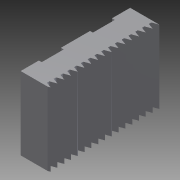
# Autodesk Inventor part: rack2
Saved by Autodesk Inventor 2011 (Build 150239000, 239)
## iProperties
Created: 2011-11-27
Part Number: rack2
Document SubType Name: Modeling
Designer: Tom
Density: 1 g/cm^3
Author: Tom
Autodesk Inventor part; units mm, degrees
ref_plane "YZ Plane" through (0, 0, 0) normal (1, 0, 0) x (0, 1, 0)
ref_plane "XZ Plane" through (0, 0, 0) normal (0, 1, 0) x (-1, 0, 0)
ref_plane "XY Plane" through (0, 0, 0) normal (0, 0, 1) x (1, 0, 0)
sketch "Sketch1" plane through (0, 0, 0) normal (0, 0, 1) x (1, 0, 0)
  line L0 (-0.515, 0.509) -> (-4.515, 0.509)
  line L1 (-4.515, -14.491) -> (-0.515, -14.491)
  line L2 (-0.515, -14.491) -> (-0.515, 0.509)
  line L3 (-4.515, -1.991) -> (-4.126, -1.991)
  line L4 (-4.126, -1.991) -> (-4.126, -4.981)
  line L5 (-4.126, -4.981) -> (-4.515, -4.981)
  line L6 (-4.515, -4.981) -> (-4.515, -1.991)
  line L7 (-4.515, -8.981) -> (-4.126, -8.981)
  line L8 (-4.126, -8.981) -> (-4.126, -11.991)
  line L9 (-4.126, -11.991) -> (-4.515, -11.991)
  line L10 (-4.515, -11.991) -> (-4.515, -8.981)
  line L11 (-4.515, 0.509) -> (-4.515, -1.991)
  line L12 (-4.515, -4.981) -> (-4.515, -14.491)
  point P0 (0, 0)
  dimension "d0" = 4
  dimension "d1" = 15
  dimension "d2" = 0.389
  dimension "d3" = 2.99
  dimension "d4" = 4
  dimension "d5" = 2.5
  dimension "d6" = 3.01
  constraints: 26 end point, 8 parallel, 4 perpendicular, 3 horizontal, 1 point on line
  measures "d0" distance of L1.start L1.end
  measures "d1" distance of L1.end L0.start
  measures "d2" distance of L3.start L3.end
  measures "d3" distance of L3.end L4.end
  measures "d4" distance between parallel lines of L7 L5
  measures "d5" distance between parallel lines of L3 L0
  measures "d6" distance of L7.end L8.end
extrude "Extrusion1" add sketch "Sketch1" along normal blind 10 contours L2 L1 L12 L9 L8 L7 L5 L4 L3 L11 L0
sketch "Sketch6" plane through (0, 0, 10) normal (0, 0, 1) x (1, 0, 0)
  line L0 (-0.515, 0.509) -> (-0.515, -14.491) projected
  line L1 (-0.515, -0.4166) -> (-1.3203, -0.1235)
  line L2 (-1.3203, -0.1235) -> (-1.3203, 0.0462)
  line L3 (-1.3203, 0.2159) -> (-0.515, 0.509)
  line L4 (-1.3203, 0.2159) -> (-1.3203, 0.0462)
  line L5 (-0.515, 0.509) -> (-0.515, -0.4166)
  line L6 (-0.412, -0.4191) -> (-1.6665, -0.4191) construction
  line L7 (-1.3203, -1.0542) -> (-0.515, -1.3473)
  line L8 (-0.515, -1.3473) -> (-0.515, -0.4216)
  line L9 (-1.3203, -1.0542) -> (-1.3203, -0.8845)
  line L10 (-1.3203, -0.7148) -> (-1.3203, -0.8845)
  line L11 (-0.515, -0.4216) -> (-1.3203, -0.7148)
  line L12 (-0.1629, -1.3498) -> (-1.5742, -1.3498) construction
  line L13 (-1.3203, -2.9154) -> (-0.515, -3.2085)
  line L14 (-0.515, -3.2085) -> (-0.515, -2.2829)
  line L15 (-1.3203, -2.9154) -> (-1.3203, -2.7457)
  line L16 (-1.3203, -2.576) -> (-1.3203, -2.7457)
  line L17 (-0.515, -2.2829) -> (-1.3203, -2.576)
  line L18 (-1.3203, -1.6454) -> (-0.515, -1.3523)
  line L19 (-0.515, -1.3523) -> (-0.515, -2.2779)
  line L20 (-1.3203, -1.6454) -> (-1.3203, -1.8151)
  line L21 (-1.3203, -1.9848) -> (-1.3203, -1.8151)
  line L22 (-0.515, -2.2779) -> (-1.3203, -1.9848)
  line L23 (-0.071, -3.211) -> (-1.4404, -3.211) construction
  line L24 (-1.3203, -6.6379) -> (-0.515, -6.9311)
  line L25 (-0.515, -6.9311) -> (-0.515, -6.0054)
  line L26 (-1.3203, -6.6379) -> (-1.3203, -6.4682)
  line L27 (-1.3203, -6.2985) -> (-1.3203, -6.4682)
  line L28 (-0.515, -6.0054) -> (-1.3203, -6.2985)
  line L29 (-1.3203, -5.3679) -> (-0.515, -5.0748)
  line L30 (-0.515, -5.0748) -> (-0.515, -6.0004)
  line L31 (-1.3203, -5.3679) -> (-1.3203, -5.5376)
  line L32 (-1.3203, -5.7073) -> (-1.3203, -5.5376)
  line L33 (-0.515, -6.0004) -> (-1.3203, -5.7073)
  line L34 (-1.3203, -3.5067) -> (-0.515, -3.2135)
  line L35 (-0.515, -3.2135) -> (-0.515, -4.1392)
  line L36 (-1.3203, -3.5067) -> (-1.3203, -3.6764)
  line L37 (-1.3203, -3.846) -> (-1.3203, -3.6764)
  line L38 (-0.515, -4.1392) -> (-1.3203, -3.846)
  line L39 (-0.515, -4.1442) -> (-1.3203, -4.4373)
  line L40 (-0.515, -5.0698) -> (-0.515, -4.1442)
  line L41 (-1.3203, -4.7767) -> (-0.515, -5.0698)
  line L42 (-1.3203, -4.7767) -> (-1.3203, -4.607)
  line L43 (-1.3203, -4.4373) -> (-1.3203, -4.607)
  line L44 (0.2425, -6.9336) -> (-1.3203, -6.9336) construction
  line L45 (-1.3203, -8.4992) -> (-0.515, -8.7923)
  line L46 (-0.515, -8.7923) -> (-0.515, -7.8667)
  line L47 (-0.515, -7.8667) -> (-1.3203, -8.1598)
  line L48 (-1.3203, -8.1598) -> (-1.3203, -8.3295)
  line L49 (-1.3203, -8.4992) -> (-1.3203, -8.3295)
  line L50 (-1.3203, -7.2292) -> (-0.515, -6.9361)
  line L51 (-1.3203, -7.2292) -> (-1.3203, -7.3989)
  line L52 (-1.3203, -7.5686) -> (-1.3203, -7.3989)
  line L53 (-0.515, -7.8617) -> (-1.3203, -7.5686)
  line L54 (-0.515, -6.9361) -> (-0.515, -7.8617)
  line L55 (-1.3203, -10.9517) -> (-0.515, -10.6586)
  line L56 (-0.515, -10.6586) -> (-0.515, -11.5842)
  line L57 (-1.3203, -10.9517) -> (-1.3203, -11.1214)
  line L58 (-1.3203, -11.2911) -> (-1.3203, -11.1214)
  line L59 (-0.515, -11.5842) -> (-1.3203, -11.2911)
  line L60 (-0.515, -9.7279) -> (-1.3203, -10.0211)
  line L61 (-1.3203, -10.0211) -> (-1.3203, -10.1908)
  line L62 (-1.3203, -10.3605) -> (-1.3203, -10.1908)
  line L63 (-1.3203, -10.3605) -> (-0.515, -10.6536)
  line L64 (-0.515, -10.6536) -> (-0.515, -9.7279)
  line L65 (-0.515, -8.7973) -> (-0.515, -9.7229)
  line L66 (-0.515, -9.7229) -> (-1.3203, -9.4298)
  line L67 (-1.3203, -9.0904) -> (-1.3203, -9.2601)
  line L68 (-1.3203, -9.4298) -> (-1.3203, -9.2601)
  line L69 (-1.3203, -9.0904) -> (-0.515, -8.7973)
  line L70 (-4.515, -8.981) -> (-4.515, -4.981) projected
  line L71 (0.0056, -11.5867) -> (-1.782, -11.5867) construction
  line L72 (-1.3203, -16.5355) -> (-0.515, -16.2424)
  line L73 (-1.3203, -16.5355) -> (-1.3203, -16.7052)
  line L74 (-1.3203, -16.8749) -> (-1.3203, -16.7052)
  line L75 (-0.515, -17.168) -> (-1.3203, -16.8749)
  line L76 (-0.515, -16.2424) -> (-0.515, -17.168)
  line L77 (-0.515, -15.3117) -> (-1.3203, -15.6048)
  line L78 (-1.3203, -15.6048) -> (-1.3203, -15.7745)
  line L79 (-1.3203, -15.9442) -> (-0.515, -16.2374)
  line L80 (-1.3203, -15.9442) -> (-1.3203, -15.7745)
  line L81 (-0.515, -16.2374) -> (-0.515, -15.3117)
  line L82 (-0.515, -14.3811) -> (-0.515, -15.3067)
  line L83 (-0.515, -15.3067) -> (-1.3203, -15.0136)
  line L84 (-1.3203, -15.0136) -> (-1.3203, -14.8439)
  line L85 (-1.3203, -14.6742) -> (-1.3203, -14.8439)
  line L86 (-1.3203, -14.6742) -> (-0.515, -14.3811)
  line L87 (-1.3203, -14.083) -> (-0.515, -14.3761)
  line L88 (-1.3203, -14.083) -> (-1.3203, -13.9133)
  line L89 (-1.3203, -13.7436) -> (-1.3203, -13.9133)
  line L90 (-0.515, -13.4505) -> (-1.3203, -13.7436)
  line L91 (-0.515, -14.3761) -> (-0.515, -13.4505)
  line L92 (-0.515, -13.4455) -> (-1.3203, -13.1524)
  line L93 (-1.3203, -13.1524) -> (-1.3203, -12.9827)
  line L94 (-1.3203, -12.813) -> (-1.3203, -12.9827)
  line L95 (-1.3203, -12.813) -> (-0.515, -12.5198)
  line L96 (-0.515, -12.5198) -> (-0.515, -13.4455)
  line L97 (-1.3203, -12.2217) -> (-0.515, -12.5148)
  line L98 (-1.3203, -12.2217) -> (-1.3203, -12.052)
  line L99 (-1.3203, -11.8823) -> (-1.3203, -12.052)
  line L100 (-0.515, -11.5892) -> (-1.3203, -11.8823)
  line L101 (-0.515, -12.5148) -> (-0.515, -11.5892)
  dimension "d70" = 0
  dimension "d71" = 0
  dimension "d72" = 70
  dimension "d73" = 0.8053
  dimension "d74" = 70
  dimension "d76" = 0.1697
  dimension "d77" = 110
  dimension "d78" = 70
  dimension "d79" = 40
  dimension "d80" = 0.9256
  dimension "d81" = 0.0025
  dimension "d82" = 0.0025
  dimension "d83" = 0.0025
  dimension "d84" = 0.0025
  dimension "d87" = 0.0025
  constraints: 200 end point, 90 symmetric about line, 5 perpendicular
  measures "d70" distance between parallel lines of L0 L5
  measures "d71" distance of L0.start L3.end
  measures "d72" angle of L0 L3
  measures "d73" distance between parallel lines of L0 L4
  measures "d74" angle of L0 L1
  measures "d76" distance of L2.start L4.end
  measures "d77" angle of L1 L2
  measures "d78" angle of L5 L1
  measures "d79" angle of L3 L1
  measures "d80" distance of L5.end L3.end
  measures "d81" distance from line of L6 L5.end
  measures "d82" distance from line of L12 L7.end
  measures "d83" distance from line of L23 L13.end
  measures "d84" distance from line of L24.end L44
  measures "d87" distance from line of L71 L59.start
extrude "Extrusion4" cut sketch "Sketch6" against normal through all contours L0 L82 L83 L84 L85 L86 | L0 L87 L88 L89 L90 | L0 L92 L93 L94 L95 | L0 L97 L98 L99 L100 | L0 L59 L58 L57 L55 | L0 L63 L62 L61 L60 | L0 L66 L68 L67 L69 | L0 L45 L49 L48 L47 | L0 L53 L52 L51 L50 | L0 L24 L26 L27 L28 | L0 L33 L32 L31 L29 | L0 L41 L42 L43 L39 | L0 L38 L37 L36 L34 | L0 L13 L15 L16 L17 | L0 L22 L21 L20 L18 | L0 L7 L9 L10 L11 | L0 L1 L2 L4 L3
equation "\"d14\" = 15.81278"
equation "\"d15\" = 20deg"
equation "\"d16\" = 8.01181"
equation "\"d17\" = 10.54185"
equation "\"d18\" = 3.31182"
equation "\"d24\" = 15.81278"
equation "\"d25\" = 20deg"
equation "\"d26\" = 8.01181"
equation "\"d27\" = 10.54185"
equation "\"d28\" = 3.31182"
equation "\"d35\" = 15.81278"
equation "\"d36\" = 20deg"
equation "\"d37\" = 8.01181"
equation "\"d38\" = 10.54185"
equation "\"d39\" = 3.31182"
equation "\"d59\" = 3.35558"
equation "\"d60\" = 20deg"
equation "\"d61\" = 2.55024"
equation "\"d62\" = 3.35558"
equation "\"d63\" = 1.05419"
body "Solid1"
